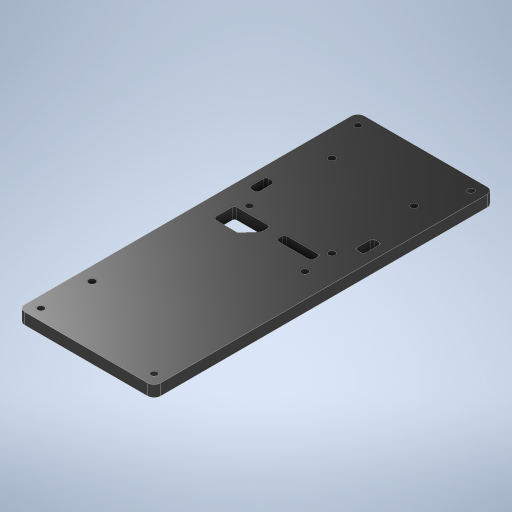
# Autodesk Inventor part: DeGiua
Saved by Autodesk Inventor 2023 (Build 270158000, 158)
## iProperties
Created: 2023-10-13
Part Number: DeGiua
Material: Generic
Document SubType Name: Modeling
Designer: Admins
Density: 1 g/cm^3
Appearance: Glossy - Black
Author: Admins
Autodesk Inventor part; units mm, degrees
ref_plane "YZ Plane" through (0, 0, 0) normal (1, 0, 0) x (0, 1, 0)
ref_plane "XZ Plane" through (0, 0, 0) normal (0, 1, 0) x (-1, 0, 0)
ref_plane "XY Plane" through (0, 0, 0) normal (0, 0, 1) x (1, 0, 0)
sketch "Sketch1" plane through (0, 0, 0) normal (0, 1, 0) x (-1, 0, 0)
  line L0 (-30, 75) -> (30, 75)
  line L1 (30, 75) -> (30, -75)
  line L2 (30, -75) -> (-30, -75)
  line L3 (-30, -75) -> (-30, 75)
  line L4 (-30, 75) -> (30, -75) construction
  line L5 (30, 75) -> (-30, -75) construction
  line L6 (30, 75) -> (25, 75)
  line L7 (25, 75) -> (25, 70)
  line L8 (25, 70) -> (30, 70)
  line L9 (30, 70) -> (30, 75)
  line L10 (-30, 75) -> (-25, 75)
  line L11 (-25, 75) -> (-25, 70)
  line L12 (-25, 70) -> (-30, 70)
  line L13 (-30, 70) -> (-30, 75)
  line L14 (30, -75) -> (25, -75)
  line L15 (25, -75) -> (25, -70)
  line L16 (25, -70) -> (30, -70)
  line L17 (30, -70) -> (30, -75)
  line L18 (-30, -75) -> (-25, -75)
  line L19 (-25, -75) -> (-25, -70)
  line L20 (-25, -70) -> (-30, -70)
  line L21 (-30, -70) -> (-30, -75)
  circle A0 centre (25, 70) radius 1.4
  circle A1 centre (-25, 70) radius 1.4
  circle A2 centre (25, -70) radius 1.4
  circle A3 centre (-25, -70) radius 1.4
  line L22 (30, -75) -> (-30, -75)
  line L23 (-30, -75) -> (-30, -55)
  line L24 (-30, -55) -> (30, -55)
  line L25 (30, -55) -> (30, -75)
  line L26 (0, -55) -> (21.5, -55)
  line L27 (21.5, -55) -> (21.5, -12)
  line L28 (21.5, -12) -> (0, -12)
  line L29 (0, -12) -> (0, -55)
  line L30 (0, -12) -> (-21.5, -12)
  line L31 (-21.5, -12) -> (-21.5, -55)
  line L32 (-21.5, -55) -> (0, -55)
  line L33 (0, -55) -> (0, -12)
  line L34 (0, -12) -> (0, -33.5)
  line L35 (-18.2, -15.3) -> (18.2, -15.3)
  line L36 (18.2, -15.3) -> (18.2, -51.7)
  line L37 (18.2, -51.7) -> (-18.2, -51.7)
  line L38 (-18.2, -51.7) -> (-18.2, -15.3)
  line L39 (-18.2, -15.3) -> (18.2, -51.7) construction
  line L40 (18.2, -15.3) -> (-18.2, -51.7) construction
  circle A4 centre (18.2, -15.3) radius 1.5
  circle A5 centre (18.2, -51.7) radius 1.5
  circle A6 centre (-18.2, -15.3) radius 1.5
  circle A7 centre (-18.2, -51.7) radius 1.5
  line L41 (-30, 75) -> (-19.18, 75)
  line L42 (-19.18, 75) -> (-19.18, -2.4)
  line L43 (-19.18, -2.4) -> (-30, -2.4)
  line L44 (-30, -2.4) -> (-30, 75)
  line L45 (30, 75) -> (24, 75)
  line L46 (24, 75) -> (24, 48.4)
  line L47 (24, 48.4) -> (30, 48.4)
  line L48 (30, 48.4) -> (30, 75)
  circle A8 centre (24, 48.4) radius 1.5
  circle A9 centre (-19.18, -2.4) radius 1.5
  line L49 (-21.5, -12) -> (-21.5, -22)
  line L50 (-21.5, -22) -> (-25.5, -22)
  line L51 (-25.5, -22) -> (-25.5, -30)
  line L52 (-25.5, -30) -> (-21.5, -30)
  line L53 (-21.5, -30) -> (-21.5, -22)
  line L54 (21.5, -22) -> (25.5, -22)
  line L55 (25.5, -22) -> (25.5, -30)
  line L56 (25.5, -30) -> (21.5, -30)
  line L57 (21.5, -30) -> (21.5, -22)
  line L58 (21.5, -12) -> (15.5, -12)
  line L59 (15.5, -12) -> (5.5, -12)
  line L60 (5.5, -12) -> (5.5, -8)
  line L61 (5.5, -8) -> (15.5, -8)
  line L62 (15.5, -8) -> (15.5, -12)
  line L63 (-21.5, -12) -> (-16.5, -12)
  line L64 (-16.5, -12) -> (-0.5, -12)
  line L65 (-0.5, -12) -> (-0.5, -8)
  line L66 (-0.5, -8) -> (-16.5, -8)
  line L67 (-16.5, -8) -> (-16.5, -12)
  line L68 (21.5, -12) -> (10.5, -12)
  line L69 (10.5, -12) -> (10.5, -2.4)
  line L70 (10.5, -2.4) -> (21.5, -2.4)
  line L71 (21.5, -2.4) -> (21.5, -12)
  line L72 (5.5, -8) -> (10.5, -2.4)
  point P0 (10.5, -8)
  dimension "d10" = 60
  dimension "d11" = 150
  dimension "d12" = 5
  dimension "d13" = 5
  dimension "d14" = 5
  dimension "d15" = 5
  dimension "d16" = 5
  dimension "d17" = 5
  dimension "d18" = 5
  dimension "d19" = 5
  dimension "d20" = 2.8
  dimension "d21" = 2.8
  dimension "d22" = 2.8
  dimension "d23" = 2.8
  dimension "d28" = 20
  dimension "d29" = 21.5
  dimension "d30" = 43
  dimension "d31" = 21.5
  dimension "d32" = 36.4
  dimension "d33" = 36.4
  dimension "d34" = 3
  dimension "d35" = 3
  dimension "d36" = 3
  dimension "d37" = 3
  dimension "d38" = 10.82
  dimension "d39" = 77.4
  dimension "d40" = 6
  dimension "d41" = 26.6
  dimension "d42" = 3
  dimension "d43" = 3
  dimension "d48" = 10
  dimension "d49" = 4
  dimension "d50" = 8
  dimension "d51" = 4
  dimension "d52" = 8
  dimension "d53" = 6
  dimension "d54" = 10
  dimension "d55" = 4
  dimension "d56" = 5
  dimension "d57" = 16
  dimension "d58" = 4
  constraints: 146 end point, 32 parallel, 16 horizontal, 16 perpendicular, 10 centre point, 10 coincident, 6 point on line, 4 midpoint
  measures "d10" distance of L1.end L2.end
  measures "d11" distance of L0.end L1.end
  measures "d12" distance of L8.end L7.end
  measures "d13" distance of L7.end L6.end
  measures "d14" distance of L11.end L12.end
  measures "d15" distance of L10.end L11.end
  measures "d16" distance of L15.end L16.end
  measures "d17" distance of L14.end L15.end
  measures "d18" distance of L20.end L19.end
  measures "d19" distance of L19.end L18.end
  measures "d20" diameter of A0
  measures "d21" diameter of A1
  measures "d22" diameter of A2
  measures "d23" diameter of A3
  measures "d28" distance of L22.end L23.end
  measures "d29" distance of L28.end L27.end
  measures "d30" distance of L27.end L26.end
  measures "d31" distance of L32.end L31.end
  measures "d32" distance of L36.end L37.end
  measures "d33" distance of L35.end L36.end
  measures "d34" diameter of A4
  measures "d35" diameter of A5
  measures "d36" diameter of A6
  measures "d37" diameter of A7
  measures "d38" distance of L42.end L43.end
  measures "d39" distance of L41.end L42.end
  measures "d40" distance of L47.end L46.end
  measures "d41" distance of L46.end L45.end
  measures "d42" diameter of A8
  measures "d43" diameter of A9
  measures "d48" distance of L30.end L49.end
  measures "d49" distance of L52.end L51.end
  measures "d50" distance of L51.end L50.end
  measures "d51" distance of L55.end L56.end
  measures "d52" distance of L54.end L55.end
  measures "d53" distance of L27.end L58.end
  measures "d54" distance of L60.end L61.end
  measures "d55" distance of L59.end L60.end
  measures "d56" distance of L30.end L63.end
  measures "d57" distance of L66.end L65.end
  measures "d58" distance of L65.end L64.end
extrude "Extrusion1" add sketch "Sketch1" along normal blind 5 contours L0 L11 A1 L12 L3 | L0 L42 A9 L43 L3 L12 A1 L11 | L0 L46 A0 A8 L47 L1 L24 L27 L56 L55 L54 L71 L70 L72 L60 L28 L30 L65 L66 L67 L31 L50 L51 L52 L3 L43 A9 L42 | L0 L7 A0 L46 | A9 L43 L42 | L42 L43 A9 | L24 L1 L16 A2 L15 L2 L19 A3 L20 L3 | L0 L1 L8 A0 L7 | L20 A3 L19 L2 L3 | L31 L30 L29 L35 A6 L38 A7 L37 L24 | A0 L8 L1 L47 A8 L46 | L29 L37 A5 L36 A4 L35 L28 L27 L24 | L52 L51 L50 L31 | A8 L47 L46 | L46 L47 A8 | L37 A7 L38 A6 L35 L29 | L29 L35 A4 L36 A5 L37 | L15 A2 L16 L1 L2 | L27 L54 L55 L56 | A5 L36 L37 | L37 L36 A5 | A7 L38 L37 | L37 L38 A7 | L67 L66 L65 L30 | L28 L62 L61 L69 L70 L71 | A6 L38 L35 | L35 L38 A6 | A4 L36 L35 | L35 L36 A4 | L28 L69 L61 L62 | L60 L61 L69 L28 | L69 L61 L72
fillet "Fillet1" radius 2.8 1 edges at (30, 2.5, 75)
fillet "Fillet2" radius 2.8 3 edges at (-30, 2.5, 75) (-30, 2.5, -75) (30, 2.5, -75)
extrude "Extrusion2" cut sketch "Sketch1" along normal blind 10 contours A8 L47 L46 | L46 L47 A8 | A5 L36 L37 | L37 L36 A5 | A7 L38 L37 | L37 L38 A7 | A6 L38 L35 | L35 L38 A6 | A4 L36 L35 | L35 L36 A4
extrude "Extrusion3" cut sketch "Sketch1" along normal blind 10 contours A9 L43 L42 | L42 L43 A9
extrude "Extrusion4" cut sketch "Sketch1" along normal blind 10 contours L52 L51 L50 L31 | L27 L54 L55 L56 | L67 L66 L65 L30 | L28 L69 L61 L62 | L60 L61 L69 L28
extrude "Extrusion5" cut sketch "Sketch1" along normal blind 10 contours L28 L62 L61 L69 L70 L71
extrude "Extrusion6" cut sketch "Sketch1" along normal blind 10 contours L69 L61 L72
fillet "Fillet3" radius 1 17 edges at (-5.5, 2.5, -8) (-10.5, 2.5, -2.4) (-21.5, 2.5, -2.4) (-21.5, 2.5, -12) (-5.5, 2.5, -12) (0.5, 2.5, -8) (0.5, 2.5, -12) (16.5, 2.5, -12) (16.5, 2.5, -8) (25.5, 2.5, -22) (21.5, 2.5, -22) (25.5, 2.5, -30) (21.5, 2.5, -30) (-25.5, 2.5, -30) (-25.5, 2.5, -22) (-21.5, 2.5, -22) (-21.5, 2.5, -30)
body "Solid1"
